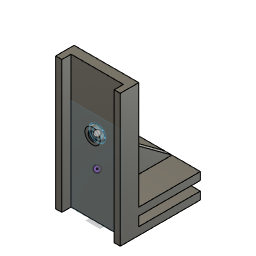
support odo main v1 (Autodesk Fusion 360 design; units mm, degrees)
Autodesk Fusion 360 part; units mm, degrees
note: some values were not read from the file. Chosen so that the rebuilt part matches the saved one: which face or edge a step refers to; where a thread starts.
sketch "Sketch1" plane through (0, 0, 0) normal (0, 0, 1) x (1, 0, 0)
  line L0 (-10.5, -15) -> (10.5, -15)
  line L1 (10.5, -15) -> (10.5, 15)
  line L2 (10.5, 15) -> (-10.5, 15)
  line L3 (-10.5, 15) -> (-10.5, -15)
  line L4 (-10.5, -15) -> (10.5, 15) construction
  line L5 (10.5, -15) -> (-10.5, 15) construction
  dimension "d1" = 21
  dimension "d2" = 30
  constraint perpendicular L0 L1
  constraint parallel L0 L2
  constraint parallel L1 L3
  constraint horizontal L0
  constraint coincident L4 origin
  constraint coincident L5 origin
  measures "d1" distance of L1.end L2.end
  measures "d2" distance of L0.end L1.end
extrude "Extrude1" add sketch "Sketch1" along normal blind 3
sketch "Sketch2" plane through (0, 0, 3) normal (0, 0, 1) x (1, 0, 0)
  line L0 (-10.5, 15) -> (-10.5, -15)
  line L1 (-10.5, -15) -> (10.5, -15)
  line L2 (10.5, -15) -> (10.5, 15)
  line L3 (10.5, 15) -> (-10.5, 15)
  line L4 (-10.5, 15) -> (-8.5, 15)
  line L5 (-8.5, 15) -> (-8.5, -15)
  line L6 (-8.5, -15) -> (-10.5, -15)
  line L7 (-10.5, -15) -> (-10.5, 15)
  line L8 (10.5, 15) -> (8.5, 15)
  line L9 (8.5, 15) -> (8.5, -15)
  line L10 (8.5, -15) -> (10.5, -15)
  line L11 (10.5, -15) -> (10.5, 15)
  dimension "d5" = 2
  dimension "d6" = 2
  constraint horizontal L4
  constraint vertical L5
  constraint horizontal L6
  constraint vertical L7
  constraint coincident L0.start L3.end
  constraint horizontal L8
  constraint vertical L9
  constraint horizontal L10
  constraint vertical L11
  constraint coincident L2.end L3.start
  measures "d5" distance of L0.start L4.end
  measures "d6" distance of L2.end L8.end
extrude "Extrude2" add sketch "Sketch2" along normal blind 3 contours L0 L1 L3 L4 L5 L6 L7 | L1 L2 L3 L8 L9 L10 L11
sketch "Sketch3" plane through (0, 0, 3) normal (0, 0, 1) x (1, 0, 0)
  line L0 (8.5, -15) -> (8.5, 15)
  line L1 (8.5, 15) -> (-8.5, 15)
  line L2 (-8.5, 15) -> (-8.5, -15)
  line L3 (-8.5, -15) -> (8.5, -15)
  circle A0 centre (0, 10) radius 1.5
  circle A1 centre (0, 10) radius 2.5
  dimension "d9" = 3
  dimension "d10" = 5
  dimension "d19" = 25
  dimension "d20" = 25
  measures "d9" diameter of A0
  measures "d10" diameter of A1
  measures "d19" distance of L3 A0.centre
  measures "d20" distance of L3 A0.centre
extrude "Extrude6" add 1 faces at (2.8333, 15, 1) along direction (0, 1, 0) blind 13
extrude "Extrude3" add sketch "Sketch3" along normal blind 1.5 contours A0 | A1
sketch "Sketch4" plane through (0, 0, 4.5) normal (0, 0, 1) x (1, 0, 0)
  circle A0 centre (0, 10) radius 2.5
  circle A1 centre (0, 10) radius 1.5
  dimension "d13" = 3
  constraint concentric A0 A1
  measures "d13" diameter of A1
extrude "Extrude4" cut sketch "Sketch4" against normal blind 6 contours A1
extrude "Extrude5" add 1 faces at (-2.8333, -15, 1) along direction (0, 1, 0) blind 13
sketch "Sketch5" plane through (0, 0, 0) normal (0, 0, -1) x (-1, 0, 0)
  line L0 (-10.5, 28) -> (-10.5, -15)
  line L1 (-10.5, -15) -> (10.5, -15)
  line L2 (10.5, -15) -> (10.5, 28)
  line L3 (10.5, 28) -> (-10.5, 28)
  circle A0 centre (0, 10) radius 1.5
  line L4 (-10.5, -15) -> (10.5, -15)
  line L5 (10.5, -15) -> (10.5, -12.5)
  line L6 (10.5, -12.5) -> (-10.5, -12.5)
  line L7 (-10.5, -12.5) -> (-10.5, -15)
  line L8 (-10.5, -9.5) -> (10.5, -9.5)
  line L9 (10.5, -9.5) -> (10.5, -7)
  line L10 (10.5, -7) -> (-10.5, -7)
  line L11 (-10.5, -7) -> (-10.5, -9.5)
  dimension "d23" = 2.5
  dimension "d24" = 2.5
  dimension "d25" = 3
  constraint horizontal L4
  constraint vertical L5
  constraint horizontal L6
  constraint vertical L7
  constraint coincident L0.end L1.start
  constraint horizontal L8
  constraint vertical L9
  constraint horizontal L10
  constraint vertical L11
  constraint coincident L0 L8.start
  measures "d23" distance of L0.end L6.end
  measures "d24" distance of L8.start L10.end
  measures "d25" distance of L6 L8
extrude "Extrude7" add sketch "Sketch5" along normal blind 20 contours L0 L2 L8 L9 L10 L11 | L0 L1 L2 L4 L5 L6 L7
sketch "Sketch6" plane through (0, 0, 0) normal (0, 0, -1) x (-1, 0, 0)
  line L0 (-10.5, -7) -> (10.5, -7)
  line L1 (10.5, -7) -> (10.5, 28)
  line L2 (10.5, 28) -> (-10.5, 28)
  line L3 (-10.5, 28) -> (-10.5, -7)
  circle A0 centre (0, 10) radius 1.5
  line L4 (1.25, -7.7426) -> (-1.25, -7.7426)
  line L5 (-1.25, -7.7426) -> (-1.25, 7.7426)
  line L6 (-1.25, 7.7426) -> (1.25, 7.7426)
  line L7 (1.25, 7.7426) -> (1.25, -7.7426)
  line L8 (1.25, -7.7426) -> (-1.25, 7.7426) construction
  line L9 (-1.25, -7.7426) -> (1.25, 7.7426) construction
  dimension "d28" = 2.5
  constraint perpendicular L4 L5
  constraint parallel L4 L6
  constraint parallel L5 L7
  constraint horizontal L4
  constraint coincident L8 origin
  constraint coincident L9 origin
  measures "d28" distance of L5.end L6.end
extrude "Extrude8" add sketch "Sketch6" along normal blind 20 contours L0 L5 L6 L7
sketch "Sketch7" plane through (-1.25, 0, 0) normal (-1, 0, 0) x (0, 0, 1)
  line L0 (0, -7) -> (0, 7.7426)
  line L1 (0, 7.7426) -> (-20, 7.7426)
  line L2 (-20, 7.7426) -> (-20, -7)
  line L3 (-20, -7) -> (0, -7)
  line L4 (-20, -7) -> (0, 7.7426)
  constraint coincident L2.end L3.start
  constraint coincident L0.end L1.start
extrude "Extrude9" cut sketch "Sketch7" against normal blind 5 contours L1 L2 L4
thread "Thread1" "ISO Metric profile 3.0 M3x0.5 6H" major diameter 3.086 minor diameter 2.529 pitch 0.5 angle 60 modelled right hand crest width 0.1368 on face at (1.4925, 9.8506, 3) crest through (1.2645, 10, 0.375)
named bodies: "support odo main"
